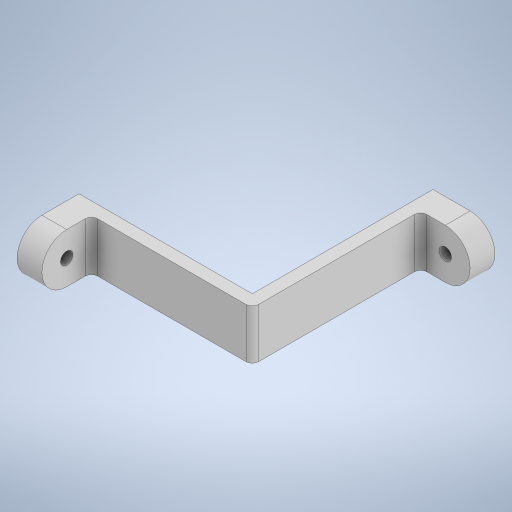
# Autodesk Inventor part: Battery mount top
Saved by Autodesk Inventor 2024 (Build 280153000, 153)
## iProperties
Created: 2023-08-08
Part Number: Battery mount top
Material: Generic
Document SubType Name: Modeling
Designer: 18179
Density: 1 g/cm^3
Appearance: Default
Author: 18179
Autodesk Inventor part; units mm, degrees
ref_plane "YZ Plane" through (0, 0, 0) normal (1, 0, 0) x (0, 1, 0)
ref_plane "XZ Plane" through (0, 0, 0) normal (0, 1, 0) x (-1, 0, 0)
ref_plane "XY Plane" through (0, 0, 0) normal (0, 0, 1) x (1, 0, 0)
sketch "Sketch1" plane through (0, 0, 0) normal (0, 1, 0) x (-1, 0, 0)
  line L0 (0, 0) -> (86.36, 0)
  line L1 (86.36, 0) -> (86.36, -180.34)
  line L2 (86.36, -180.34) -> (0, -180.34)
  line L3 (0, -180.34) -> (0, 0)
  line L4 (-2.4049, 2.4049) -> (88.7649, 2.4049)
  line L5 (88.7649, 2.4049) -> (88.7649, -182.7449)
  line L6 (88.7649, -182.7449) -> (-2.4049, -182.7449)
  line L7 (-2.4049, -182.7449) -> (-2.4049, 2.4049)
  line L8 (-8.7549, 8.7549) -> (95.1149, 8.7549)
  line L9 (95.1149, 8.7549) -> (95.1149, -189.0949)
  line L10 (95.1149, -189.0949) -> (-8.7549, -189.0949)
  line L11 (-8.7549, -189.0949) -> (-8.7549, 8.7549)
  line L12 (86.36, 0) -> (86.36, 48.8454)
  line L13 (86.36, 48.8454) -> (86.36, -245.5667)
  line L14 (86.36, 8.7549) -> (73.66, 8.7549)
  line L15 (73.66, 8.7549) -> (73.66, 34.1549)
  line L16 (73.66, 34.1549) -> (86.36, 34.1549)
  line L17 (86.36, 34.1549) -> (86.36, 8.7549)
  line L18 (86.36, -189.0949) -> (73.66, -189.0949)
  line L19 (73.66, -189.0949) -> (73.66, -214.4949)
  line L20 (73.66, -214.4949) -> (86.36, -214.4949)
  line L21 (86.36, -214.4949) -> (86.36, -189.0949)
  point P0 (86.36, 34.1549)
  point P1 (73.66, 8.7549)
  point P2 (73.66, -189.0949)
  point P3 (86.36, -214.4949)
  point P4 (86.36, -182.7449)
  point P5 (86.36, 2.4049)
  dimension "d0" = 86.36
  dimension "d1" = 180.34
  dimension "d2" = 6.35
  dimension "d3" = 12.7
  dimension "d4" = 25.4
  dimension "d5" = 12.7
  dimension "d6" = 25.4
  constraints: 44 end point, 10 parallel, 6 perpendicular, 5 point on line, 3 horizontal, 6 other
  measures "d0" distance of L1.end L2.end
  measures "d1" distance of L0.end L1.end
  measures "d2" distance between parallel lines of L7 L11
  measures "d3" distance of L15.end L16.end
  measures "d4" distance of L14.end L15.end
  measures "d5" distance of L20.end L19.end
  measures "d6" distance of L19.end L18.end
extrude "Extrusion1" add sketch "Sketch1" along normal blind 25.4 contours L4 L7 L6 L13 L10 L11 L8 L12 | L8 L15 L16 L12 | L13 L20 L19 L10
fillet "Fillet1" radius 3.175 4 edges at (8.7549, 12.7, 8.7549) (8.7549, 12.7, -189.0949) (-73.66, 12.7, 8.7549) (-73.66, 12.7, -189.0949)
fillet "Fillet2" radius 12.7 4 edges at (-80.01, 25.4, 34.1549) (-80.01, 0, 34.1549) (-80.01, 25.4, -214.4949) (-80.01, 0, -214.4949)
sketch "Sketch2" plane through (-73.66, 0, -192.2699) normal (1, 0, 0) x (0, 0, -1)
  arc A0 (-213.7248, 25.4) -> (-213.7248, 0) centre (-213.7248, 12.7) ccw projected
  line L0 (-213.7248, 0) -> (-204.1998, 0) projected
  line L1 (-204.1998, 25.4) -> (-204.1998, 0) projected
  line L2 (-213.7248, 25.4) -> (-204.1998, 25.4) projected
  arc A1 (9.525, 0) -> (9.525, 25.4) centre (9.525, 12.7) ccw projected
  line L3 (0, 25.4) -> (9.525, 25.4) projected
  line L4 (0, 0) -> (0, 25.4) projected
  line L5 (0, 0) -> (9.525, 0) projected
  circle A2 centre (-213.7248, 12.7) radius 3.175
  circle A3 centre (9.525, 12.7) radius 3.175
  point P0 (-192.2699, 0)
  dimension "d11" = 6.35
  dimension "d12" = 6.35
  constraints: 2 centre point, 2 coincident
  measures "d11" diameter of A2
  measures "d12" diameter of A3
extrude "Extrusion2" cut sketch "Sketch2" against normal blind 25.4 contours A2 | A3
sketch "Sketch3" plane through (8.7549, 0, 5.5799) normal (1, 0, 0) x (0, 0, -1)
  line L0 (0, 25.4) -> (191.4998, 25.4) projected
  line L1 (95.7499, 25.4) -> (95.7499, 0)
  line L2 (188.3248, 0) -> (3.175, 0) projected
  line L3 (83.0499, 25.4) -> (83.0499, 0)
  point P0 (5.5799, 0)
  point P1 (83.0499, 0)
  dimension "d15" = 12.7
  constraints: 4 end point, 2 midpoint, 1 parallel
  measures "d15" distance between parallel lines of L1 L3
extrude "Extrusion3" add sketch "Sketch3" along normal blind 25.4
sketch "Sketch4" plane through (8.7549, 0, -185.9199) normal (1, 0, 0) x (0, 0, -1)
  line L0 (-3.175, 25.4) -> (-188.3248, 25.4) projected
  line L1 (-95.7499, 25.4) -> (115.4033, 25.4)
  line L2 (115.4033, 25.4) -> (115.4033, -38.5479)
  line L3 (115.4033, -38.5479) -> (-95.7499, -38.5479)
  line L4 (-95.7499, -38.5479) -> (-95.7499, 25.4)
  point P0 (-185.9199, 0)
  point P1 (-3.175, 25.4)
  constraints: 8 end point, 2 parallel, 1 horizontal, 1 midpoint, 1 perpendicular
extrude "Extrusion4" cut sketch "Sketch4" along normal through all both and the other way through all
fillet "Fillet3" radius 12.7 2 edges at (34.1549, 25.4, -83.82) (34.1549, 0, -83.82)
fillet "Fillet4" radius 3.175 1 edges at (8.7549, 12.7, -77.47)
sketch "Sketch5" plane through (21.4549, 12.7, -77.47) normal (0, 0, 1) x (1, 0, 0)
  arc A0 (0, -12.7) -> (0, 12.7) centre (0, 0) ccw projected
  circle A1 centre (0, 0) radius 3.175
  point P0 (-21.4549, -12.7)
  dimension "d22" = 6.35
  constraints: 1 centre point, 1 coincident
  measures "d22" diameter of A1
extrude "Extrusion5" cut sketch "Sketch5" against normal blind 25.4
body "Solid1"
